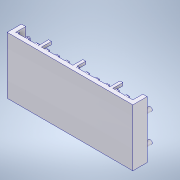
# Autodesk Inventor part: grip_4
Saved by Autodesk Inventor 2020 (Build 240168000, 168)
## iProperties
Created: 2019-10-09
Part Number: grip_4
Material: Generic
Document SubType Name: Modeling
Designer: ayad493
Density: 1 g/cm^3
Appearance: Cool White
Author: ayad493
Autodesk Inventor part; units mm, degrees
ref_plane "YZ Plane" through (0, 0, 0) normal (1, 0, 0) x (0, 1, 0)
ref_plane "XZ Plane" through (0, 0, 0) normal (0, 1, 0) x (-1, 0, 0)
ref_plane "XY Plane" through (0, 0, 0) normal (0, 0, 1) x (1, 0, 0)
sketch "Sketch1" plane through (0, 0, 0) normal (0, 0, 1) x (1, 0, 0)
  circle A0 centre (0, 0) radius 4
  arc A1 (0, 8) -> (0, -8) centre (0, 0) ccw
  circle A2 centre (60, 0) radius 4
  arc A3 (60, -8) -> (60, 8) centre (60, 0) ccw
  line L0 (0, 0) -> (4, 0)
  line L1 (60, 0) -> (45, 0)
  line L2 (15, 0) -> (15, -3.325)
  line L3 (45, 0) -> (45, -3.325)
  circle A4 centre (15, -1.6625) radius 1.6625
  circle A5 centre (45, -1.6625) radius 1.6625
  line L4 (0, -8) -> (60, -8)
  line L5 (0, 0) -> (0, 4)
  line L6 (0, 8) -> (30, 0)
  line L7 (30, 0) -> (60, 8)
  line L8 (0, 0) -> (15, 0)
  line L9 (45, 0) -> (60, 0)
  dimension "d0" = 8
  dimension "d1" = 16
  dimension "d2" = 60
  dimension "d3" = 8
  dimension "d4" = 16
  dimension "d5" = 3.325
  dimension "d63" = 60
  constraints: 20 end point, 6 point on circle, 4 centre point, 4 coincident, 3 horizontal, 2 midpoint, 2 vertical, 2 vertical alignment, 1 perpendicular, 1 tangent, 4 other
  measures "d0" diameter of A0
  measures "d1" diameter of A1
  measures "d2" distance of L0.start L9.end
  measures "d3" diameter of A2
  measures "d4" diameter of A3
  measures "d5" distance of L2.start L2.end
  measures "d63" distance of L4.start L4.end
extrude "Extrusion1" add sketch "Sketch1" along normal blind 20
fillet "Fillet2" radius 2 1 edges at (30, 0, 10)
sketch "Sketch20" plane through (0, -8, 0) normal (0, -1, 0) x (1, 0, 0)
  line L0 (60, 0) -> (60, 20) projected
  line L1 (60, 10) -> (52, 10)
  line L2 (52, 10) -> (52, 15)
  line L3 (-8, 0) -> (-8, 20) projected
  line L4 (52, 15) -> (-8, 15)
  line L5 (-8, 15) -> (-8, 5)
  line L6 (-8, 5) -> (52, 5)
  line L7 (52, 5) -> (52, 15)
  point P0 (0, 0)
  dimension "d65" = 5
  constraints: 12 end point, 2 horizontal, 2 parallel, 2 perpendicular, 1 midpoint, 1 point on line
  measures "d65" distance of L1.end L2.end
extrude "Extrusion18" cut sketch "Sketch20" against normal blind 20
sketch "Sketch21" plane through (0, -8, 0) normal (0, -1, 0) x (1, 0, 0)
  line L0 (0, 15) -> (0, 20) projected
  line L1 (0, 15) -> (8, 15)
  line L2 (-4, 15) -> (4, 15) projected
  line L3 (8, 15) -> (8, 5)
  line L4 (52, 5) -> (0, 5) projected
  line L5 (8, 15) -> (52, 15)
  line L6 (52, 15) -> (52, 5)
  line L7 (52, 5) -> (8, 5)
  line L8 (8, 5) -> (8, 15)
  constraints: 12 end point, 3 equal length, 2 perpendicular, 1 horizontal
extrude "Extrusion20" add sketch "Sketch21" against normal blind 4
sketch "Sketch22" plane through (0, 0, 20) normal (0, 0, 1) x (1, 0, 0)
  line L0 (52, -4) -> (8, -4) projected
  line L1 (8, -4) -> (10, -4)
  line L2 (10, -8) -> (10, -4)
  line L3 (10, -4) -> (10, -5)
  line L4 (10, -5) -> (52, -5)
  line L5 (52, -5) -> (52, -7)
  line L6 (52, -7) -> (10, -7)
  line L7 (10, -7) -> (10, -5)
  point P0 (0, 0)
  constraints: 14 end point, 2 parallel, 2 perpendicular, 2 point on line, 1 horizontal
extrude "Extrusion21" cut sketch "Sketch22" against normal blind 20
sketch "Sketch23" plane through (0, -8, 0) normal (0, -1, 0) x (1, 0, 0)
  line L0 (8, 5) -> (52, 5) projected
  line L1 (52, 15) -> (8, 15) projected
  line L2 (8, 15) -> (8, 5)
  line L3 (8, 5) -> (8, 15) projected
  circle A0 centre (13.5, 7.5) radius 1.5
  circle A1 centre (13.5, 12.5) radius 1.5
  circle A2 centre (23.5, 7.5) radius 1.5
  circle A3 centre (23.5, 12.5) radius 1.5
  circle A4 centre (33.5, 7.5) radius 1.5
  circle A5 centre (33.5, 12.5) radius 1.5
  circle A6 centre (43.5, 7.5) radius 1.5
  circle A7 centre (43.5, 12.5) radius 1.5
  line L4 (13.5, 12.5) -> (13.5, 17.5)
  line L5 (13.3375, 15) -> (13.3375, 20) projected
  line L6 (12, 16) -> (15, 16)
  line L7 (15, 16) -> (15, 19)
  line L8 (15, 19) -> (12, 19)
  line L9 (12, 19) -> (12, 16)
  line L10 (12, 16) -> (15, 19) construction
  line L11 (15, 16) -> (12, 19) construction
  line L12 (25, 19) -> (22, 19)
  line L13 (25, 16) -> (25, 19)
  line L14 (22, 19) -> (22, 16)
  line L15 (22, 16) -> (25, 16)
  line L16 (35, 19) -> (32, 19)
  line L17 (35, 16) -> (35, 19)
  line L18 (32, 19) -> (32, 16)
  line L19 (32, 16) -> (35, 16)
  line L20 (45, 19) -> (42, 19)
  line L21 (45, 16) -> (45, 19)
  line L22 (42, 19) -> (42, 16)
  line L23 (42, 16) -> (45, 16)
  line L24 (15, 14) -> (12, 14)
  line L25 (15, 11) -> (15, 14)
  line L26 (12, 14) -> (12, 11)
  line L27 (12, 11) -> (15, 11)
  line L28 (25, 14) -> (22, 14)
  line L29 (25, 11) -> (25, 14)
  line L30 (22, 14) -> (22, 11)
  line L31 (22, 11) -> (25, 11)
  line L32 (35, 14) -> (32, 14)
  line L33 (35, 11) -> (35, 14)
  line L34 (32, 14) -> (32, 11)
  line L35 (32, 11) -> (35, 11)
  line L36 (45, 14) -> (42, 14)
  line L37 (45, 11) -> (45, 14)
  line L38 (42, 14) -> (42, 11)
  line L39 (42, 11) -> (45, 11)
  line L40 (15, 9) -> (12, 9)
  line L41 (15, 6) -> (15, 9)
  line L42 (12, 9) -> (12, 6)
  line L43 (12, 6) -> (15, 6)
  line L44 (25, 9) -> (22, 9)
  line L45 (25, 6) -> (25, 9)
  line L46 (22, 9) -> (22, 6)
  line L47 (22, 6) -> (25, 6)
  line L48 (35, 9) -> (32, 9)
  line L49 (35, 6) -> (35, 9)
  line L50 (32, 9) -> (32, 6)
  line L51 (32, 6) -> (35, 6)
  line L52 (45, 9) -> (42, 9)
  line L53 (45, 6) -> (45, 9)
  line L54 (42, 9) -> (42, 6)
  line L55 (42, 6) -> (45, 6)
  line L56 (15, 4) -> (12, 4)
  line L57 (15, 1) -> (15, 4)
  line L58 (12, 4) -> (12, 1)
  line L59 (12, 1) -> (15, 1)
  line L60 (25, 4) -> (22, 4)
  line L61 (25, 1) -> (25, 4)
  line L62 (22, 4) -> (22, 1)
  line L63 (22, 1) -> (25, 1)
  line L64 (35, 4) -> (32, 4)
  line L65 (35, 1) -> (35, 4)
  line L66 (32, 4) -> (32, 1)
  line L67 (32, 1) -> (35, 1)
  line L68 (45, 4) -> (42, 4)
  line L69 (45, 1) -> (45, 4)
  line L70 (42, 4) -> (42, 1)
  line L71 (42, 1) -> (45, 1)
  point P0 (0, 0)
  dimension "d76" = 5
  dimension "d79" = 10
  dimension "d172" = 5
  dimension "d174" = 3
  dimension "d175" = 3
  dimension "d178" = 10
  dimension "d181" = 5
  constraints: 136 end point, 8 centre point, 3 horizontal, 3 parallel, 2 midpoint, 2 vertical, 1 perpendicular, 134 other
  measures "d76" distance of A0.centre L4.start
  measures "d79" distance of A0.centre A2.centre
  measures "d172" distance of L4.start L4.end
  measures "d174" distance of L8.end L7.end
  measures "d175" distance of L7.end L6.end
  measures "d178" distance of L7.end L12.start
  measures "d181" distance of L7.end L24.start
sketch "Sketch24" plane through (0, -8, 0) normal (0, -1, 0) x (1, 0, 0)
  circle A0 centre (13.5, 7.5) radius 1.5 projected
  circle A1 centre (23.5, 12.5) radius 1.5 projected
  line L0 (13.5, 7.5) -> (23.5, 12.5)
  circle A2 centre (33.5, 7.5) radius 1.5 projected
  line L1 (23.5, 12.5) -> (33.5, 7.5)
  circle A3 centre (43.5, 12.5) radius 1.5 projected
  line L2 (33.5, 7.5) -> (43.5, 12.5)
  line L3 (20, 8.5) -> (17, 8.5)
  line L4 (17, 8.5) -> (17, 11.5)
  line L5 (17, 11.5) -> (20, 11.5)
  line L6 (20, 11.5) -> (20, 8.5)
  line L7 (20, 8.5) -> (17, 11.5) construction
  line L8 (17, 8.5) -> (20, 11.5) construction
  line L9 (27, 8.5) -> (30, 8.5)
  line L10 (30, 8.5) -> (30, 11.5)
  line L11 (30, 11.5) -> (27, 11.5)
  line L12 (27, 11.5) -> (27, 8.5)
  line L13 (27, 8.5) -> (30, 11.5) construction
  line L14 (30, 8.5) -> (27, 11.5) construction
  line L15 (40, 8.5) -> (37, 8.5)
  line L16 (37, 8.5) -> (37, 11.5)
  line L17 (37, 11.5) -> (40, 11.5)
  line L18 (40, 11.5) -> (40, 8.5)
  line L19 (40, 8.5) -> (37, 11.5) construction
  line L20 (37, 8.5) -> (40, 11.5) construction
  circle A4 centre (13.5, 12.5) radius 1.5 projected
  line L21 (13.5, 7.5) -> (13.5, 12.5)
  line L22 (13.5, 12.5) -> (13.5, 20)
  line L23 (13.5, 15) -> (13.5, 20)
  line L24 (0, 20) -> (60, 20) projected
  line L25 (12, 16) -> (15, 16)
  line L26 (15, 16) -> (15, 19)
  line L27 (15, 19) -> (12, 19)
  line L28 (12, 19) -> (12, 16)
  line L29 (12, 16) -> (15, 19) construction
  line L30 (15, 16) -> (12, 19) construction
  line L31 (12, 4) -> (12, 1)
  line L32 (12, 1) -> (15, 1)
  line L33 (15, 1) -> (15, 4)
  line L34 (15, 4) -> (12, 4)
  line L35 (22, 19) -> (22, 16)
  line L36 (22, 16) -> (25, 16)
  line L37 (25, 16) -> (25, 19)
  line L38 (25, 19) -> (22, 19)
  line L39 (22, 4) -> (22, 1)
  line L40 (22, 1) -> (25, 1)
  line L41 (25, 1) -> (25, 4)
  line L42 (25, 4) -> (22, 4)
  line L43 (32, 19) -> (32, 16)
  line L44 (32, 16) -> (35, 16)
  line L45 (35, 16) -> (35, 19)
  line L46 (35, 19) -> (32, 19)
  line L47 (32, 4) -> (32, 1)
  line L48 (32, 1) -> (35, 1)
  line L49 (35, 1) -> (35, 4)
  line L50 (35, 4) -> (32, 4)
  line L51 (42, 19) -> (42, 16)
  line L52 (42, 16) -> (45, 16)
  line L53 (45, 16) -> (45, 19)
  line L54 (45, 19) -> (42, 19)
  line L55 (42, 4) -> (42, 1)
  line L56 (42, 1) -> (45, 1)
  line L57 (45, 1) -> (45, 4)
  line L58 (45, 4) -> (42, 4)
  point P0 (0, 0)
  point P1 (18.5, 10)
  point P2 (28.5, 10)
  point P3 (38.5, 10)
  point P4 (13.5, 17.5)
  dimension "d84" = 3
  dimension "d85" = 3
  dimension "d88" = 15
  dimension "d91" = 10
  constraints: 116 end point, 12 midpoint, 9 parallel, 5 horizontal, 5 perpendicular, 4 point on line, 2 vertical, 56 other
  measures "d84" distance of L3.end L4.end
  measures "d85" distance of L16.end L17.end
  measures "d88" distance of L27.end L31.start
  measures "d91" distance of L27.end L35.start
extrude "Extrusion23" add sketch "Sketch24" against normal blind 4 contours L4 L5 L6 L0 | L0 L6 L3 L4 | L12 L11 L10 L1 | L1 L10 L9 L12 | L16 L17 L18 L2 | L2 L18 L15 L16 | L25 L28 L27 L22 | L22 L27 L26 L25 | L34 L33 L32 L31 | L38 L37 L36 L35 | L42 L41 L40 L39 | L46 L45 L44 L43 | L50 L49 L48 L47 | L54 L53 L52 L51 | L58 L57 L56 L55
sketch "Sketch25" plane through (0, -8, 0) normal (0, -1, 0) x (1, 0, 0)
  line L0 (68, 0) -> (68, 20) projected
  line L1 (68, 0) -> (52, 0)
  line L2 (52, 0) -> (52, 6)
  line L3 (52, 6) -> (68, 6)
  line L4 (68, 6) -> (68, 0)
  line L5 (68, 20) -> (60, 20) projected
  line L6 (68, 20) -> (52, 20)
  line L7 (52, 20) -> (52, 14)
  line L8 (52, 14) -> (68, 14)
  line L9 (68, 14) -> (68, 20)
  point P0 (0, 0)
  constraints: 16 end point, 4 parallel, 2 horizontal, 2 perpendicular, 2 point on line
extrude "Extrusion24" cut sketch "Sketch25" against normal blind 18
sketch "Sketch26" plane through (0, -8, 15) normal (0, -1, 0) x (1, 0, 0)
  line L0 (52, -15) -> (30.5153, -15) projected
  line L1 (52, -15) -> (50, -15)
  line L2 (50, -15) -> (50, 5)
  line L3 (50, 5) -> (52, 5)
  line L4 (52, 5) -> (52, -15)
  point P0 (0, -15)
  constraints: 8 end point, 2 parallel, 1 horizontal, 1 perpendicular
extrude "Extrusion25" add sketch "Sketch26" against normal blind 16
sketch "Sketch27" plane through (0, 0, 0) normal (0, 0, -1) x (-1, 0, 0)
  line L0 (-52, -8) -> (-52, 5.8667) projected
  line L1 (-50, -4) -> (-50, 5.3333) projected
  line L2 (-52, 5.8667) -> (-50, 5.3333)
  line L3 (-50, 5.3333) -> (-50, 8)
  line L4 (-52, 8) -> (-50, 8) projected
  line L5 (-50, 8) -> (-52, 8)
  line L6 (-52, 8) -> (-52, 5.8667)
  line L7 (-52, 8) -> (-52, -8) projected
  point P0 (0, 0)
  constraints: 8 end point, 3 collinear
extrude "Extrusion26" cut sketch "Sketch27" against normal blind 20
fillet "Fillet3" radius 2 3 edges at (60, 8, 10) (0, 8, 2.5) (0, 8, 17.5)
sketch "Sketch28" plane through (60, -8, 6) normal (0, 0, -1) x (-1, 0, 0)
  line L0 (0, 0) -> (8, 0) projected
  line L1 (0, 0) -> (0, 1)
  circle A0 centre (15, 6.3375) radius 1.6625 projected
  line L2 (15, 6.3375) -> (15, 8)
  arc A1 (-0.3247, 15.9934) -> (0, 0) centre (0, 8) ccw projected
  arc A2 (-5.6569, 13.6569) -> (5, 1.755) centre (0, 8) ccw
  line L3 (10, 5.0386) -> (5, 1.755)
  arc A3 (-4.773, 12.773) -> (4.1504, 2.6768) centre (0, 8) ccw
  line L4 (15, 8) -> (15, 9.5)
  line L5 (15, 9.5) -> (4.1504, 2.6768)
  line L6 (10, 4) -> (10, 13.3333) projected
  line L7 (10, 6.3555) -> (10, 5.0386)
  line L8 (-4.773, 12.773) -> (-5.6569, 13.6569)
  line L9 (0, 8) -> (8, 8) construction
  line L10 (8, 0) -> (0, 0) projected
  line L11 (0, 0) -> (8, 0)
  line L12 (8, 0) -> (8, 3.7252)
  line L13 (8, 13.8667) -> (8, 0) projected
  point P0 (60, 8)
  dimension "d103" = 13.5
  dimension "d104" = 1.5
  dimension "d105" = 135
  constraints: 20 end point, 5 point on circle, 5 point on line, 3 vertical, 2 centre point, 2 coincident, 1 collinear, 1 horizontal, 1 vertical alignment, 1 other
  measures "d103" diameter of A3
  measures "d104" distance of L2.end L4.end
  measures "d105" angle of L9 L8
extrude "Extrusion29" cut sketch "Sketch28" against normal blind 5 contours A2 L3 L12 L0 | A1 L8 A3 L5 L13 L3 A2 | L13 L5 L6 L3
sketch "Sketch30" plane through (52, -2.9022, 6) normal (0, 0, -1) x (-1, 0, 0)
  circle A0 centre (-8, 2.9022) radius 4 projected
  arc A1 (-13.6569, 8.5591) -> (-8, -5.0978) centre (-8, 2.9022) ccw
  arc A2 (-12.773, 7.6752) -> (-3.8496, -2.421) centre (-8, 2.9022) ccw
  line L0 (0, -5.0978) -> (0, 8.7689) projected
  line L1 (-3.8496, -2.421) -> (2, 1.2578) projected
  line L2 (0, 0) -> (-0.7447, -0.4683)
  line L3 (-8, -5.0978) -> (0, -5.0978) projected
  line L4 (0, 0) -> (0, -5.0978)
  line L5 (0, -5.0978) -> (-8, -5.0978)
  line L6 (-13.6569, 8.5591) -> (-12.773, 7.6752) projected
  line L7 (-12.773, 7.6752) -> (-13.6569, 8.5591)
  line L8 (0, -1.3726) -> (0, 0) projected
  line L9 (0, -1.3726) -> (2, -0.0592) projected
  line L10 (0, -1.3726) -> (2, -0.0592)
  line L11 (2, 1.2578) -> (2, -0.0592) projected
  line L12 (2, -0.0592) -> (2, 1.2578)
  line L13 (2, 1.2578) -> (0, 0) projected
  line L14 (2, 1.2578) -> (0, 0)
  line L15 (0, 0) -> (0, -1.3726)
  point P0 (52, 2.9022)
  constraints: 18 end point, 6 collinear, 5 point on circle, 4 point on line, 2 centre point, 2 coincident, 1 vertical
extrude "Extrusion33" add sketch "Sketch30" against normal blind 3 contours L6 A2 L1 L0 L3 A1 | L0 L1 L11 L9
fillet "Fillet4" radius 2 1 edges at (64.773, 4.773, 10)
fillet "Fillet5" radius 2 1 edges at (52, -4.2748, 10)
sketch "Sketch31" plane through (0, -8, 15) normal (0, -1, 0) x (1, 0, 0)
  line L0 (52, -15) -> (52, -9) projected
  line L1 (10, 5) -> (10, -15) projected
  line L2 (52, -15) -> (10, -15)
  line L3 (10, -15) -> (10, -12)
  line L4 (10, -12) -> (52, -12)
  line L5 (52, -12) -> (52, -15)
  line L6 (52, 5) -> (10, 5)
  line L7 (10, 5) -> (10, 2)
  line L8 (10, 2) -> (52, 2)
  line L9 (52, 2) -> (52, 5)
  point P0 (0, -15)
  constraints: 16 end point, 4 parallel, 3 point on line, 2 horizontal, 2 perpendicular
extrude "Extrusion34" add sketch "Sketch31" against normal blind 3
sketch "Sketch32" plane through (8, -8, 5) normal (-1, 0, 0) x (0, 0, 1)
  line L0 (6, 1.25) -> (4, 1.25) projected
  line L1 (6, 2.6459) -> (4, 2.6459) projected
  line L2 (6, 1.25) -> (4, 2.6459)
  circle A0 centre (5, 1.9479) radius 0.75
  point P0 (-5, 8)
  dimension "d124" = 1.5
  constraints: 2 end point, 1 centre point, 1 midpoint, 1 point on line
  measures "d124" diameter of A0
extrude "Extrusion35" cut sketch "Sketch32" against normal blind 3 contours A0 L0 | L0 A0 L2 | L2 A0 L1 | A0 L1 picked at (5.0916, 1.7153) picked at (5.0915, 2.1806)
sketch "Sketch33" plane through (0, 0, 20) normal (0, 0, 1) x (1, 0, 0)
  line L0 (0, -8) -> (52, -8) projected
  line L1 (8, -8) -> (8, -14)
  line L2 (8, -14) -> (50, -14)
  line L3 (52, -12) -> (52, -8)
  line L4 (52, -8) -> (51.5, -8)
  line L5 (51.5, -8) -> (51.5, -10.5)
  line L6 (49.5, -12.5) -> (8.5, -12.5) construction
  line L7 (8.5, -12.5) -> (8.5, -8)
  arc A0 (49.5, -12.5) -> (51.5, -10.5) centre (49.5, -10.5) ccw
  arc A1 (50, -14) -> (52, -12) centre (50, -12) ccw
  line L8 (49, -12) -> (49.5, -12.5)
  line L9 (49, -12) -> (48.5, -12.5)
  line L10 (48.5, -12.5) -> (48, -12)
  line L11 (48, -12) -> (47.5, -12.5)
  line L12 (47, -12) -> (47.5, -12.5)
  line L13 (47, -12) -> (46.5, -12.5)
  line L14 (46.5, -12.5) -> (46, -12)
  line L15 (46, -12) -> (45.5, -12.5)
  line L16 (45, -12) -> (45.5, -12.5)
  line L17 (45, -12) -> (44.5, -12.5)
  line L18 (44.5, -12.5) -> (44, -12)
  line L19 (44, -12) -> (43.5, -12.5)
  line L20 (43, -12) -> (43.5, -12.5)
  line L21 (43, -12) -> (42.5, -12.5)
  line L22 (42.5, -12.5) -> (42, -12)
  line L23 (42, -12) -> (41.5, -12.5)
  line L24 (41, -12) -> (41.5, -12.5)
  line L25 (41, -12) -> (40.5, -12.5)
  line L26 (40.5, -12.5) -> (40, -12)
  line L27 (40, -12) -> (39.5, -12.5)
  line L28 (39, -12) -> (39.5, -12.5)
  line L29 (39, -12) -> (38.5, -12.5)
  line L30 (38.5, -12.5) -> (38, -12)
  line L31 (38, -12) -> (37.5, -12.5)
  line L32 (37, -12) -> (37.5, -12.5)
  line L33 (37, -12) -> (36.5, -12.5)
  line L34 (36.5, -12.5) -> (36, -12)
  line L35 (36, -12) -> (35.5, -12.5)
  line L36 (35, -12) -> (35.5, -12.5)
  line L37 (35, -12) -> (34.5, -12.5)
  line L38 (34.5, -12.5) -> (34, -12)
  line L39 (34, -12) -> (33.5, -12.5)
  line L40 (33, -12) -> (33.5, -12.5)
  line L41 (33, -12) -> (32.5, -12.5)
  line L42 (32.5, -12.5) -> (32, -12)
  line L43 (32, -12) -> (31.5, -12.5)
  line L44 (31, -12) -> (31.5, -12.5)
  line L45 (31, -12) -> (30.5, -12.5)
  line L46 (30.5, -12.5) -> (30, -12)
  line L47 (30, -12) -> (29.5, -12.5)
  line L48 (29, -12) -> (29.5, -12.5)
  line L49 (29, -12) -> (28.5, -12.5)
  line L50 (28.5, -12.5) -> (28, -12)
  line L51 (28, -12) -> (27.5, -12.5)
  line L52 (27, -12) -> (27.5, -12.5)
  line L53 (27, -12) -> (26.5, -12.5)
  line L54 (26.5, -12.5) -> (26, -12)
  line L55 (26, -12) -> (25.5, -12.5)
  line L56 (25, -12) -> (25.5, -12.5)
  line L57 (25, -12) -> (24.5, -12.5)
  line L58 (24.5, -12.5) -> (24, -12)
  line L59 (24, -12) -> (23.5, -12.5)
  line L60 (23, -12) -> (23.5, -12.5)
  line L61 (23, -12) -> (22.5, -12.5)
  line L62 (22.5, -12.5) -> (22, -12)
  line L63 (22, -12) -> (21.5, -12.5)
  line L64 (21, -12) -> (21.5, -12.5)
  line L65 (21, -12) -> (20.5, -12.5)
  line L66 (20.5, -12.5) -> (20, -12)
  line L67 (20, -12) -> (19.5, -12.5)
  line L68 (19, -12) -> (19.5, -12.5)
  line L69 (19, -12) -> (18.5, -12.5)
  line L70 (18.5, -12.5) -> (18, -12)
  line L71 (18, -12) -> (17.5, -12.5)
  line L72 (17, -12) -> (17.5, -12.5)
  line L73 (17, -12) -> (16.5, -12.5)
  line L74 (16.5, -12.5) -> (16, -12)
  line L75 (16, -12) -> (15.5, -12.5)
  line L76 (15, -12) -> (15.5, -12.5)
  line L77 (15, -12) -> (14.5, -12.5)
  line L78 (14.5, -12.5) -> (14, -12)
  line L79 (14, -12) -> (13.5, -12.5)
  line L80 (13, -12) -> (13.5, -12.5)
  line L81 (13, -12) -> (12.5, -12.5)
  line L82 (12.5, -12.5) -> (12, -12)
  line L83 (12, -12) -> (11.5, -12.5)
  line L84 (11, -12) -> (11.5, -12.5)
  line L85 (11, -12) -> (10.5, -12.5)
  line L86 (10.5, -12.5) -> (10, -12)
  line L87 (10, -12) -> (9.5, -12.5)
  line L88 (49.5, -12.5) -> (49, -12)
  line L89 (48.5, -12.5) -> (48, -12)
  line L90 (47.5, -12.5) -> (47, -12)
  line L91 (46.5, -12.5) -> (46, -12)
  line L92 (45.5, -12.5) -> (45, -12)
  line L93 (44.5, -12.5) -> (44, -12)
  line L94 (43.5, -12.5) -> (43, -12)
  line L95 (42.5, -12.5) -> (42, -12)
  line L96 (41.5, -12.5) -> (41, -12)
  line L97 (40.5, -12.5) -> (40, -12)
  line L98 (39.5, -12.5) -> (39, -12)
  line L99 (38.5, -12.5) -> (38, -12)
  line L100 (38, -12) -> (37.5, -12.5)
  line L101 (37, -12) -> (36.5, -12.5)
  line L102 (36, -12) -> (35.5, -12.5)
  line L103 (35, -12) -> (34.5, -12.5)
  line L104 (34, -12) -> (33.5, -12.5)
  line L105 (33, -12) -> (32.5, -12.5)
  line L106 (32, -12) -> (31.5, -12.5)
  line L107 (31, -12) -> (30.5, -12.5)
  line L108 (30, -12) -> (29.5, -12.5)
  line L109 (29, -12) -> (28.5, -12.5)
  line L110 (28, -12) -> (27.5, -12.5)
  line L111 (27, -12) -> (26.5, -12.5)
  line L112 (26, -12) -> (25.5, -12.5)
  line L113 (25, -12) -> (24.5, -12.5)
  line L114 (24, -12) -> (23.5, -12.5)
  line L115 (23, -12) -> (22.5, -12.5)
  line L116 (22, -12) -> (21.5, -12.5)
  line L117 (21, -12) -> (20.5, -12.5)
  line L118 (20, -12) -> (19.5, -12.5)
  line L119 (19, -12) -> (18.5, -12.5)
  line L120 (18, -12) -> (17.5, -12.5)
  line L121 (17, -12) -> (16.5, -12.5)
  line L122 (16, -12) -> (15.5, -12.5)
  line L123 (15, -12) -> (14.5, -12.5)
  line L124 (14, -12) -> (13.5, -12.5)
  line L125 (13, -12) -> (12.5, -12.5)
  line L126 (12, -12) -> (11.5, -12.5)
  line L127 (11, -12) -> (10.5, -12.5)
  line L128 (10, -12) -> (9.5, -12.5)
  line L129 (9.5, -12.5) -> (8.5, -12.5)
  line L130 (52, -8) -> (51.5, -8)
  line L131 (8.5, -8) -> (8, -8)
  line L132 (52, -8) -> (52, 5.8667) projected
  line L133 (52, -12) -> (52, -8)
  line L134 (52, -8) -> (51.5, -8)
  line L135 (52, -8) -> (51.5, -8)
  line L136 (9.5, -12.5) -> (8.5, -12.5)
  line L137 (8.5, -14) -> (49.5, -14)
  line L138 (49.5, -14) -> (49.5, -12.5)
  arc A2 (50, -14) -> (52, -12) centre (50, -12) ccw
  line L139 (8, -14) -> (8.5, -14)
  line L140 (8.5, -12.5) -> (8.5, -8)
  line L141 (8.5, -8) -> (8, -8)
  line L142 (8, -8) -> (8, -14)
  line L143 (0, -8) -> (52, -8) projected
  line L144 (51.5, -8) -> (52, -8)
  line L145 (52, -8) -> (52, -12)
  line L146 (51.5, -8) -> (51.5, -10.5)
  point P0 (0, 0)
  point P1 (51.5, -12.5)
  dimension "d129" = 43
  dimension "d130" = 2
  dimension "d134" = 2
  dimension "d139" = 0.5
  dimension "d140" = 0.5
  dimension "d158" = 4.5
  dimension "d159" = 6
  dimension "d160" = 2.5
  constraints: 289 end point, 32 collinear, 22 coincident, 14 perpendicular, 12 parallel, 6 point on circle, 6 point on line, 5 horizontal, 5 tangent, 3 centre point, 1 equal radius, 1 vertical, 190 other
  measures "d129" distance of L6.end point (51.5, -12.5)
  measures "d130" radius of A0
  measures "d134" distance of L6.start point (47.5, -12.5)
  measures "d139" horizontal distance of L9.end L8.start
  measures "d140" horizontal distance of L9.end L10.end
  measures "d158" distance of L6.end L7.end
  measures "d159" distance of L1.start L1.end
  measures "d160" distance of L4.end L5.end
extrude "Extrusion36" add sketch "Sketch33" against normal blind 20 contours L0 L7 L129 L87 L86 L85 L84 L83 L82 L81 L80 L79 L78 L77 L76 L75 L74 L73 L72 L71 L70 L69 L68 L67 L66 L65 L64 L63 L62 L61 L60 L59 L58 L57 L56 L55 L54 L53 L52 L51 L50 L49 L48 L47 L46 L45 L44 L43 L42 L41 L40 L39 L38 L37 L36 L35 L34 L33 L32 L31 L30 L29 L28 L27 L26 L25 L24 L23 L22 L21 L20 L19 L18 L17 L16 L15 L14 L13 L12 L11 L10 L9 L8 L138 L2 L1
sketch "Sketch35" plane through (0, 0, 20) normal (0, 0, 1) x (1, 0, 0)
  line L0 (52, 5.8667) -> (52, -8) projected
  line L1 (52, -8) -> (51.5, -8)
  line L2 (51.5, -8) -> (51.5, -14)
  line L3 (51.5, -14) -> (52, -14)
  line L4 (52, -14) -> (52, -8)
  line L5 (49.5, -14) -> (8, -14) projected
  line L6 (49.5, -14) -> (52, -14)
  line L7 (52, -14) -> (52, -13.5)
  line L8 (52, -13.5) -> (49.5, -13.5)
  line L9 (49.5, -13.5) -> (49.5, -14)
  point P0 (0, 0)
  point P1 (51.5, -13.5)
  dimension "d143" = 0.5
  dimension "d144" = 0.5
  dimension "d161" = 6
  constraints: 16 end point, 4 parallel, 2 horizontal, 2 perpendicular, 1 point on line
  measures "d143" distance of L3.end L2.end
  measures "d144" distance of L7.end L6.end
  measures "d161" distance of L3.end L0.end
sketch "Sketch36" plane through (8, -8, 0) normal (-1, 0, 0) x (0, 0, 1)
  line L0 (0, -1.5) -> (1.4518, -1.5)
  circle A0 centre (10, 1.9479) radius 0.75 projected
  line L1 (1.4518, -1.5) -> (10, -1.5)
  circle A1 centre (10, 1.9479) radius 0.75 projected
  line L2 (10, 1.9479) -> (10, -1.5)
  line L3 (10, -1.5) -> (10, -2)
  circle A2 centre (10, -2) radius 1.75
  point P0 (0, 8)
  dimension "d166" = 0.5
  dimension "d167" = 3.5
  constraints: 8 end point, 2 vertical, 1 centre point, 1 coincident, 1 horizontal
  measures "d166" distance of L1.end L3.end
  measures "d167" diameter of A2
sketch "Sketch37" plane through (0, 0, 20) normal (0, 0, 1) x (1, 0, 0)
  circle A0 centre (0, 0) radius 4
  circle A1 centre (0, 0) radius 3
  dimension "d150" = 6
  constraints: 2 centre point, 2 coincident
  measures "d150" diameter of A1
extrude "Extrusion39" add sketch "Sketch37" against normal blind 5
sketch "Sketch38" plane through (0, 0, 0) normal (0, 0, -1) x (-1, 0, 0)
  circle A0 centre (0, 0) radius 4
  circle A1 centre (0, 0) radius 3
  constraints: 2 centre point, 2 coincident
extrude "Extrusion40" add sketch "Sketch38" against normal blind 5
sketch "Sketch39" plane through (60, -8, 6) normal (0, 0, -1) x (-1, 0, 0)
  circle A0 centre (0, 8) radius 4 projected
  circle A1 centre (0, 8) radius 4
  circle A2 centre (0, 8) radius 3
  point P0 (60, 8)
  dimension "d155" = 6
  constraints: 2 centre point, 2 coincident
  measures "d155" diameter of A2
extrude "Extrusion41" add sketch "Sketch39" against normal up to surface (8 mm away)
extrude "Extrusion42" add sketch "Sketch35" against normal up to surface (20 mm away)
fillet "Fillet7" radius 3 2 edges at (52, -14, 10) (51.5, -13.5, 10)
extrude "Extrusion43" cut sketch "Sketch36" against normal blind 2 contours A2 L2 L1 | L1 L2 A2
sketch "Sketch40" plane through (0, 0, 0) normal (0, 0, -1) x (-1, 0, 0)
  line L0 (-49.5, -12.5) -> (-49, -12) projected
  line L1 (-49.5, -12.5) -> (-50.8784, -12.5)
  arc A0 (-51.5, -10.6716) -> (-49.5, -13.5) centre (-48.5, -10.6716) ccw projected
  line L2 (-49.5, -13.5) -> (-49.5, -12.5)
  arc A1 (-50.8784, -12.5) -> (-49.5, -13.5) centre (-48.5, -10.6716) ccw
  point P0 (0, 0)
  constraints: 4 end point, 3 point on circle, 1 centre point, 1 concentric, 1 horizontal, 1 perpendicular
extrude "Extrusion44" add sketch "Sketch40" against normal up to surface (20 mm away)
extrude "Extrusion45" cut sketch "Sketch23" against normal blind 2 contours L6 L5 L8 L7 | L6 L9 L8 L5 | A0 | L41 L43 A0 | A0 L40 L41 | A0 L42 L40 | L43 L42 A0 | A1 | L25 L27 A1 | A1 L24 L25 | A1 L26 L24 | L27 L26 A1 | A2 | L45 L47 A2 | A2 L44 L45 | A2 L46 L44 | L47 L46 A2 | A3 | L29 L31 A3 | A3 L28 L29 | A3 L30 L28 | L31 L30 A3 | A4 | L49 L51 A4 | A4 L48 L49 | A4 L50 L48 | L51 L50 A4 | A5 | L33 L35 A5 | A5 L32 L33 | A5 L34 L32 | L35 L34 A5 | A6 | L53 L55 A6 | A6 L52 L53 | A6 L54 L52 | L55 L54 A6 | A7 | L37 L39 A7 | A7 L36 L37 | A7 L38 L36 | L39 L38 A7 | L13 L15 L14 L12 | L17 L19 L18 L16 | L21 L23 L22 L20 | L57 L59 L58 L56 | L61 L63 L62 L60 | L65 L67 L66 L64 | L69 L71 L70 L68
sketch "Sketch41" plane through (0, 0, 20) normal (0, 0, 1) x (1, 0, 0)
  line L0 (8.5, -8) -> (51.5, -8) projected
  line L1 (51.5, -8) -> (8.5, -8)
  line L2 (8.5, -12.5) -> (8.5, -8) projected
  line L3 (8.5, -8) -> (8.5, -12.5)
  line L4 (8.5, -12.5) -> (8.5, -10.25)
  line L5 (51.5, -10.25) -> (8.5, -10.25)
  line L6 (29.5, -8) -> (30.5, -8)
  line L7 (30.5, -8) -> (30.5, -12.5)
  line L8 (30.5, -12.5) -> (29.5, -12.5)
  line L9 (29.5, -12.5) -> (29.5, -8)
  line L10 (29.5, -8) -> (30.5, -12.5) construction
  line L11 (30.5, -8) -> (29.5, -12.5) construction
  line L12 (43, -12) -> (43, -8)
  line L13 (45, -8) -> (42, -8) projected
  line L14 (18, -12) -> (18, -8)
  line L15 (42.5, -12.5) -> (42, -12) projected
  line L16 (43.5, -8) -> (42.5, -8)
  line L17 (42.5, -8) -> (42.5, -12.5)
  line L18 (42.5, -12.5) -> (43.5, -12.5)
  line L19 (43.5, -12.5) -> (43.5, -8)
  line L20 (43.5, -8) -> (42.5, -12.5) construction
  line L21 (42.5, -8) -> (43.5, -12.5) construction
  line L22 (17.5, -12.5) -> (18, -12) projected
  line L23 (18.5, -8) -> (17.5, -8)
  line L24 (17.5, -8) -> (17.5, -12.5)
  line L25 (17.5, -12.5) -> (18.5, -12.5)
  line L26 (18.5, -12.5) -> (18.5, -8)
  line L27 (18.5, -8) -> (17.5, -12.5) construction
  line L28 (17.5, -8) -> (18.5, -12.5) construction
  point P0 (0, 0)
  point P1 (30, -10.25)
  point P2 (43, -10.25)
  point P3 (18, -10.25)
  dimension "d186" = 1
  constraints: 48 end point, 8 midpoint, 7 perpendicular, 6 parallel, 6 point on line, 4 horizontal
  measures "d186" distance of L7.end L8.end
extrude "Extrusion46" add sketch "Sketch41" against normal blind 1 contours L0 L14 L5 L24 | L0 L26 L5 L14 | L5 L14 L22 L24 | L5 L26 L25 L22 L14 | L0 L7 L5 L9 | L5 L7 L8 L9 | L0 L12 L5 L17 | L5 L19 L18 L17 | L0 L19 L5 L12
sketch "Sketch42" plane through (0, 0, 0) normal (0, 0, -1) x (-1, 0, 0)
  line L0 (-18.5, -12.5) -> (-18.5, -8) projected
  line L1 (-17.5, -12.5) -> (-17.5, -8) projected
  line L2 (-18.5, -8) -> (-17.5, -8)
  line L3 (-17.5, -8) -> (-17.5, -12.5)
  line L4 (-17.5, -12.5) -> (-18.5, -12.5)
  line L5 (-18.5, -12.5) -> (-18.5, -8)
  line L6 (-29, -12) -> (-29.5, -12.5) projected
  line L7 (-30.5, -8) -> (-30.5, -12.5) projected
  line L8 (-29.5, -12.5) -> (-30.5, -12.5)
  line L9 (-30.5, -12.5) -> (-30.5, -8)
  line L10 (-30.5, -8) -> (-29.5, -8)
  line L11 (-29.5, -8) -> (-29.5, -12.5)
  line L12 (-42, -8) -> (-45, -8) projected
  line L13 (-42.5, -12.5) -> (-43.5, -12.5)
  line L14 (-43.5, -12.5) -> (-43.5, -8)
  line L15 (-43.5, -8) -> (-42.5, -8)
  line L16 (-42.5, -8) -> (-42.5, -12.5)
  point P0 (0, 0)
  constraints: 24 end point, 6 parallel, 3 horizontal, 3 perpendicular, 1 midpoint
extrude "Extrusion47" add sketch "Sketch42" against normal blind 1
sketch "Sketch43" plane through (0, 0, 20) normal (0, 0, 1) x (1, 0, 0)
  circle A0 centre (0, 0) radius 3 projected
  line L0 (0, 0) -> (-5.6569, 5.6569)
  arc A1 (-0.3247, 7.9934) -> (0, -8) centre (0, 0) ccw projected
  line L1 (0, 0) -> (8, 0) construction
  circle A2 centre (-5.6569, 5.6569) radius 2.5
  point P0 (-3.6346, 7.1267)
  point P1 (-7.1267, 3.6346)
  dimension "d191" = 135
  dimension "d192" = 5
  constraints: 4 end point, 1 centre point, 1 coincident, 1 equal length, 1 horizontal, 1 point on circle
  measures "d191" angle of L1 L0
  measures "d192" diameter of A2
extrude "Extrusion48" add sketch "Sketch43" against normal up to surface (20 mm away) contours A1 A2
sketch "Sketch44" plane through (29.4847, 0.1374, 5) normal (0.2576627, 0.9662349, 0) x (0.9662349, -0.2576627, 0)
  line L0 (-33.8019, -10) -> (-30.8271, -10) projected
  line L1 (-33.8019, -10) -> (-38.8019, -10)
  line L2 (-38.8019, -10) -> (-38.8019, 0)
  line L3 (-38.8019, 0) -> (-33.8019, 0)
  line L4 (-33.8019, 0) -> (-33.8019, -10)
  point P0 (-28.4537, 5)
  dimension "d195" = 5
  dimension "d196" = 10
  constraints: 8 end point, 2 parallel, 1 horizontal, 1 perpendicular
  measures "d195" distance of L2.end L3.end
  measures "d196" distance of L1.end L2.end
extrude "Extrusion49" cut sketch "Sketch44" against normal blind 10
sketch "Sketch45" plane through (30.5153, 0.1374, 5) normal (-0.2576627, 0.9662349, 0) x (0.9662349, 0.2576627, 0)
  line L0 (18.6625, -1) -> (22.2355, -1) projected
  line L1 (22.2355, -1) -> (22.2355, -9)
  line L2 (31.4537, -9) -> (25.4537, -9) projected
  line L3 (22.2355, -5) -> (26.2355, -5)
  line L4 (24.8855, -2.6) -> (27.6389, -2.6309)
  line L5 (27.6389, -2.6309) -> (28.9889, -5.0309)
  line L6 (28.9889, -5.0309) -> (27.5855, -7.4)
  line L7 (27.5855, -7.4) -> (24.832, -7.3691)
  line L8 (24.832, -7.3691) -> (23.482, -4.9691)
  line L9 (23.482, -4.9691) -> (24.8855, -2.6)
  point P0 (-29.5204, 5)
  dimension "d199" = 8
  dimension "d200" = 4
  constraints: 16 end point, 1 horizontal, 1 midpoint, 1 perpendicular, 13 other
  measures "d199" distance of L0.end L1.end
  measures "d200" distance of L3.start L3.end
extrude "Extrusion50" cut sketch "Sketch45" against normal blind 1.7
sketch "Sketch46" plane through (0, 0, 20) normal (0, 0, 1) x (1, 0, 0)
  line L0 (52, -8) -> (52, 5.8667) projected
  line L1 (52, -8) -> (50.5, -8)
  line L2 (50.5, -8) -> (50.5, -14)
  line L3 (50.5, -14) -> (52, -14)
  line L4 (52, -14) -> (52, -8)
  line L5 (8, -8) -> (8, -14) projected
  line L6 (8, -14) -> (49, -14) projected
  line L7 (8, -8) -> (9.5, -8)
  line L8 (9.5, -8) -> (9.5, -14)
  line L9 (9.5, -14) -> (8, -14)
  line L10 (8, -14) -> (8, -8)
  point P0 (0, 0)
  dimension "d205" = 1.5
  dimension "d206" = 1.5
  constraints: 16 end point, 4 parallel, 2 horizontal, 2 perpendicular, 1 point on line
  measures "d205" distance of L3.end L2.end
  measures "d206" distance of L8.end L9.end
extrude "Extrusion51" add sketch "Sketch46" against normal up to surface (20 mm away)
sketch "Sketch47" plane through (0, 0, 20) normal (0, 0, 1) x (1, 0, 0)
  line L0 (52, 5.8667) -> (52, -14) projected
  line L1 (8, -8) -> (8, -14) projected
  line L2 (52, -14) -> (8, -14)
  line L3 (8, -14) -> (8, -13.3004)
  line L4 (8, -13.3004) -> (52, -13.3004)
  line L5 (52, -13.3004) -> (52, -14)
  point P0 (0, 0)
  constraints: 8 end point, 2 parallel, 1 horizontal, 1 perpendicular, 1 point on line
extrude "Extrusion52" add sketch "Sketch47" against normal up to surface (20 mm away)
sketch "Sketch48" plane through (8, -14, 20) normal (0, -1, 0) x (1, 0, 0)
  line L0 (42.5, -20) -> (42.5, 0) projected
  line L1 (44, -20) -> (0, -20) projected
  line L2 (42.5, -20) -> (44, -20)
  line L3 (44, -20) -> (43.25, -20)
  line L4 (43.25, -14.25) -> (43.25, -15.75)
  line L5 (43.25, -5.75) -> (43.25, -4.25)
  line L6 (44, 0) -> (22.5153, 0) projected
  line L7 (44, -14.25) -> (42.5, -14.25)
  line L8 (42.5, -14.25) -> (42.5, -15.75)
  line L9 (42.5, -15.75) -> (44, -15.75)
  line L10 (44, -15.75) -> (44, -14.25)
  line L11 (44, -14.25) -> (42.5, -15.75) construction
  line L12 (42.5, -14.25) -> (44, -15.75) construction
  line L13 (44, -4.25) -> (42.5, -4.25)
  line L14 (42.5, -4.25) -> (42.5, -5.75)
  line L15 (42.5, -5.75) -> (44, -5.75)
  line L16 (44, -5.75) -> (44, -4.25)
  line L17 (44, -4.25) -> (42.5, -5.75) construction
  line L18 (42.5, -4.25) -> (44, -5.75) construction
  line L19 (43.25, -15.75) -> (43.25, -14.25)
  line L20 (43.25, -5.75) -> (43.25, -4.25)
  line L21 (44, -9.25) -> (42.5, -9.25)
  line L22 (42.5, -9.25) -> (42.5, -10.75)
  line L23 (42.5, -10.75) -> (44, -10.75)
  line L24 (44, -10.75) -> (44, -9.25)
  line L25 (44, -9.25) -> (42.5, -10.75) construction
  line L26 (42.5, -9.25) -> (44, -10.75) construction
  line L27 (0, -20) -> (1.515, -20)
  line L28 (21.4847, -20) -> (-7.7282, -20) projected
  line L29 (0, -10.75) -> (0, -9.25) projected
  line L30 (1.5075, -14.25) -> (0.0075, -14.25)
  line L31 (0.0075, -14.25) -> (0.0075, -15.75)
  line L32 (0.0075, -15.75) -> (1.5075, -15.75)
  line L33 (1.5075, -15.75) -> (1.5075, -14.25)
  line L34 (-7.7282, -15) -> (21.4847, -15) projected
  line L35 (1.5075, -14.25) -> (0.0075, -15.75) construction
  line L36 (0.0075, -14.25) -> (1.5075, -15.75) construction
  line L37 (1.5075, -9.25) -> (0.0075, -9.25)
  line L38 (0.0075, -9.25) -> (0.0075, -10.75)
  line L39 (0.0075, -10.75) -> (1.5075, -10.75)
  line L40 (1.5075, -10.75) -> (1.5075, -9.25)
  line L41 (1.5075, -9.25) -> (0.0075, -10.75) construction
  line L42 (0.0075, -9.25) -> (1.5075, -10.75) construction
  line L43 (0, -10.75) -> (2, -10.75) projected
  line L44 (1.5075, -4.25) -> (0.0075, -4.25)
  line L45 (0.0075, -4.25) -> (0.0075, -5.75)
  line L46 (0.0075, -5.75) -> (1.5075, -5.75)
  line L47 (1.5075, -5.75) -> (1.5075, -4.25)
  line L48 (1.5075, -4.25) -> (0.0075, -5.75) construction
  line L49 (0.0075, -4.25) -> (1.5075, -5.75) construction
  line L50 (43.25, -15) -> (43.25, -14.25)
  line L51 (0.7575, -15.75) -> (0.7575, -14.25)
  line L52 (0.7575, -10.75) -> (0.7575, -10)
  line L53 (0.7575, -5.75) -> (0.7575, -4.25)
  line L54 (43.25, -10.75) -> (43.25, -9.25)
  line L55 (43.25, -5.75) -> (43.25, -5)
  line L56 (0.7575, -4.25) -> (0.7575, -5.75)
  line L57 (0.7575, -9.25) -> (0.7575, -10)
  line L58 (0.7575, -15.75) -> (0.7575, -14.25)
  line L59 (0.7575, -10.75) -> (0.7575, -9.25)
  line L60 (0.7575, 0) -> (0.7575, -5.75)
  line L61 (0.7575, -9.25) -> (0.7575, -10)
  point P0 (-8, -20)
  point P1 (43.25, -10)
  point P2 (0.7575, -15)
  point P3 (0.7575, -5)
  dimension "d211" = 1.5
  dimension "d212" = 1.5
  dimension "d213" = 1.5
  dimension "d214" = 1.5
  dimension "d215" = 1.5
  dimension "d216" = 1.5
  dimension "d217" = 1.5
  dimension "d218" = 1.5
  constraints: 110 end point, 29 midpoint, 14 parallel, 10 vertical, 8 perpendicular, 6 horizontal, 6 point on line, 1 collinear, 1 other
  measures "d211" distance of L8.end L7.end
  measures "d212" distance of L14.end L13.end
  measures "d213" distance of L23.end L22.end
  measures "d214" distance of L22.end L21.end
  measures "d215" distance of L32.end L31.end
  measures "d216" distance of L31.end L30.end
  measures "d217" distance of L39.end L38.end
  measures "d218" distance of L46.end L45.end
extrude "Extrusion53" cut sketch "Sketch48" against normal blind 8
sketch "Sketch49" plane through (0, 0, 20) normal (0, 0, 1) x (1, 0, 0)
  line L0 (8, -8) -> (-21.6494, -8)
  line L1 (-21.6494, -8) -> (-21.6494, 18.45)
  line L2 (-21.6494, 18.45) -> (71.4783, 18.45)
  line L3 (71.4783, 18.45) -> (71.4783, -8)
  line L4 (71.4783, -8) -> (-21.6494, -8)
  point P0 (0, 0)
  constraints: 10 end point, 4 perpendicular, 1 horizontal, 1 point on line
extrude "Extrusion54" cut sketch "Sketch49" against normal through all
sketch "Sketch50" plane through (0, 0, 0) normal (0, 0, -1) x (-1, 0, 0)
  line L0 (-9.5, -8) -> (-8.0075, -8) projected
  line L1 (-52, -8) -> (-52, -14) projected
  line L2 (-8.0075, -8) -> (-52, -8)
  line L3 (-52, -8) -> (-52, -9)
  line L4 (-52, -9) -> (-8.0075, -9)
  line L5 (-8.0075, -9) -> (-8.0075, -8)
  point P0 (0, 0)
  dimension "d223" = 1
  constraints: 8 end point, 2 parallel, 1 horizontal, 1 perpendicular, 1 point on line
  measures "d223" distance of L3.end L2.end
extrude "Extrusion55" cut sketch "Sketch50" against normal through all
sketch "Sketch51" plane through (8, -14, 20) normal (0, -1, 0) x (1, 0, 0)
  line L0 (1.5075, -5.75) -> (1.5075, -4.25) projected
  line L1 (0.0075, -4.25) -> (1.5075, -4.25) projected
  line L2 (1.5075, -5.75) -> (0.0075, -5.75)
  line L3 (0.0075, -5.75) -> (0.0075, -4.25)
  line L4 (0.0075, -4.25) -> (1.5075, -4.25)
  line L5 (1.5075, -4.25) -> (1.5075, -5.75)
  line L6 (1.5075, -10.75) -> (1.5075, -9.25) projected
  line L7 (0.0075, -9.25) -> (1.5075, -9.25) projected
  line L8 (1.5075, -10.75) -> (0.0075, -10.75)
  line L9 (0.0075, -10.75) -> (0.0075, -9.25)
  line L10 (0.0075, -9.25) -> (1.5075, -9.25)
  line L11 (1.5075, -9.25) -> (1.5075, -10.75)
  line L12 (1.5075, -15.75) -> (1.5075, -14.25) projected
  line L13 (1.5075, -14.25) -> (0.0075, -14.25)
  line L14 (0.0075, -14.25) -> (0.0075, -15.75)
  line L15 (0.0075, -15.75) -> (1.5075, -15.75)
  line L16 (1.5075, -15.75) -> (1.5075, -14.25)
  line L17 (42.5, 0) -> (42.5, -4.25) projected
  line L18 (44, -5.75) -> (42.5, -5.75) projected
  line L19 (42.5, -4.25) -> (44, -4.25)
  line L20 (44, -4.25) -> (44, -5.75)
  line L21 (44, -5.75) -> (42.5, -5.75)
  line L22 (42.5, -5.75) -> (42.5, -4.25)
  line L23 (42.5, -5.75) -> (42.5, -9.25) projected
  line L24 (44, -10.75) -> (42.5, -10.75) projected
  line L25 (42.5, -9.25) -> (44, -9.25)
  line L26 (44, -9.25) -> (44, -10.75)
  line L27 (44, -10.75) -> (42.5, -10.75)
  line L28 (42.5, -10.75) -> (42.5, -9.25)
  line L29 (42.5, -14.25) -> (44, -14.25) projected
  line L30 (44, -15.75) -> (42.5, -15.75) projected
  line L31 (42.5, -14.25) -> (44, -14.25)
  line L32 (44, -14.25) -> (44, -15.75)
  line L33 (44, -15.75) -> (42.5, -15.75)
  line L34 (42.5, -15.75) -> (42.5, -14.25)
  point P0 (-8, -20)
  constraints: 48 end point, 12 parallel, 6 horizontal, 6 perpendicular, 1 point on line
extrude "Extrusion56" add sketch "Sketch51" against normal blind 7
sketch "Sketch52" plane through (52, -14, 20) normal (1, 0, 0) x (0, 0, -1)
  line L0 (10.75, 6) -> (10.75, 5) projected
  line L1 (9.25, 6) -> (9.25, 7) projected
  line L2 (10.75, 5) -> (9.25, 5)
  line L3 (9.25, 5) -> (9.25, 7)
  line L4 (9.25, 7) -> (10.75, 7)
  line L5 (10.75, 7) -> (10.75, 5)
  point P0 (20, 14)
  constraints: 8 end point, 2 parallel, 1 horizontal, 1 perpendicular
extrude "Extrusion57" cut sketch "Sketch52" against normal through all
sketch "Sketch53" plane through (8.0075, -9, 20) normal (1, 0, 0) x (0, 0, -1)
  line L0 (0, 0) -> (0, -3.5) projected
  line L1 (0, 1) -> (9.25, 1) projected
  line L2 (0, 0) -> (4.2425, 0)
  line L3 (4.2425, 0) -> (4.2425, 1)
  line L4 (4.2425, 1) -> (0, 1)
  line L5 (0, 1) -> (0, 0)
  line L6 (14.25, 0) -> (5.75, 0) projected
  line L7 (5.75, 0) -> (9.2459, 0)
  line L8 (9.2459, 0) -> (9.2459, 1)
  line L9 (9.2459, 1) -> (5.75, 1)
  line L10 (5.75, 1) -> (5.75, 0)
  line L11 (10.75, 0) -> (9.25, 0) projected
  line L12 (10.75, 1) -> (14.25, 1) projected
  line L13 (10.75, 0) -> (14.25, 0)
  line L14 (14.25, 0) -> (14.25, 1)
  line L15 (14.25, 1) -> (10.75, 1)
  line L16 (10.75, 1) -> (10.75, 0)
  line L17 (20, -5) -> (20, 1) projected
  line L18 (20, 0) -> (15.75, 0) projected
  line L19 (20, 1) -> (15.75, 1)
  line L20 (15.75, 1) -> (15.75, 0)
  line L21 (15.75, 0) -> (20, 0)
  line L22 (20, 0) -> (20, 1)
  point P0 (20, 9)
  constraints: 32 end point, 8 parallel, 4 horizontal, 4 perpendicular, 2 point on line
extrude "Extrusion58" cut sketch "Sketch53" against normal blind 10
sketch "Sketch54" plane through (8, -14, 0) normal (-1, 0, 0) x (0, 0, 1)
  point P0 (0, 14)
sketch "Sketch55" plane through (8, -14, 0) normal (-1, 0, 0) x (0, 0, 1)
  line L0 (20, 1.5) -> (20, 5) projected
  line L1 (20, 5) -> (0, 5)
  line L2 (0, 5) -> (0, 7.2002)
  line L3 (0, 7.2002) -> (20, 7.2002)
  line L4 (20, 7.2002) -> (20, 5)
  point P0 (0, 14)
  constraints: 8 end point, 2 parallel, 1 horizontal, 1 perpendicular
extrude "Extrusion59" cut sketch "Sketch55" against normal through all
sketch "Sketch56" plane through (50.5, -9, 0) normal (0, 1, 0) x (1, 0, 0)
  line L0 (-42.5, -20) -> (1.5, -20) projected
  line L1 (1.5, -20) -> (0, -20)
  line L2 (-1, -20) -> (-1, 0) projected
  line L3 (0.75, -20) -> (0.75, 0)
  line L4 (1.5, -20) -> (1.5, 0) projected
  line L5 (0.75, -20) -> (0.75, -10)
  circle A0 centre (0.75, -15) radius 0.75
  line L6 (0, -20) -> (0, 0) projected
  line L7 (0.75, -10) -> (0.75, 0)
  line L8 (1.5, 0) -> (-42.5, 0) projected
  circle A1 centre (0.75, -5) radius 0.75
  line L9 (-41, -15.75) -> (-41, -20) projected
  line L10 (-42.5, -20) -> (-41, -20)
  line L11 (-41, -20) -> (-41.75, -20)
  line L12 (-41.75, -20) -> (-41.75, 0)
  line L13 (-41.75, -10) -> (-41.75, -20)
  line L14 (-41.75, -10) -> (-41.75, 0)
  circle A2 centre (-41.75, -15) radius 0.75
  circle A3 centre (-41.75, -5) radius 0.75
  point P0 (-50.5, 0)
  dimension "d234" = 1.5
  dimension "d235" = 1.5
  dimension "d236" = 1.5
  dimension "d237" = 1.5
  constraints: 18 end point, 8 midpoint, 4 centre point, 3 perpendicular, 2 collinear, 1 horizontal, 1 parallel, 1 point on line, 1 tangent
  measures "d234" distance of L0.end L1.end
  measures "d235" diameter of A1
  measures "d236" diameter of A2
  measures "d237" diameter of A3
extrude "Extrusion60" add sketch "Sketch56" along normal blind 1.8 contours A2 L12 | L12 A2 | A0 L3 | A3 L12 | L12 A3 | L3 A0 | A1 L3 | A1 L3
sketch "Sketch57" plane through (8, -14, 0) normal (-1, 0, 0) x (0, 0, 1)
  line L0 (20, 2) -> (0, 2) projected
  line L1 (9.25, 5) -> (10.75, 5) projected
  line L2 (10, 5) -> (10, 1.5075)
  line L3 (9.25, 1.5075) -> (10.75, 1.5075) projected
  circle A0 centre (10, 3.2537) radius 1.5
  point P0 (0, 14)
  dimension "d240" = 3
  constraints: 3 midpoint, 2 end point, 1 centre point
  measures "d240" diameter of A0
extrude "Extrusion61" cut sketch "Sketch57" against normal blind 1.8
fillet "Fillet8" radius 1 1 edges at (50.5, -12.5, 10)
sketch "Sketch58" plane through (0, 0, 20) normal (0, 0, 1) x (1, 0, 0)
  line L0 (17.5, -12.5) -> (17, -12) projected
  line L1 (17.5, -12.5) -> (9.5, -12.5)
  line L2 (9.5, -12.5) -> (9.5, -12)
  line L3 (9.5, -12) -> (17.5, -12)
  line L4 (17.5, -12) -> (17.5, -12.5)
  line L5 (18.5, -9) -> (18.5, -12.5) projected
  line L6 (29.5, -12.5) -> (29, -12) projected
  line L7 (18.5, -12) -> (29.5, -12)
  line L8 (29.5, -12) -> (29.5, -12.5)
  line L9 (29.5, -12.5) -> (18.5, -12.5)
  line L10 (18.5, -12.5) -> (18.5, -12)
  line L11 (42.5, -9) -> (42.5, -12.5) projected
  line L12 (30.5, -12) -> (42.5, -12)
  line L13 (42.5, -12) -> (42.5, -12.5)
  line L14 (42.5, -12.5) -> (30.5, -12.5)
  line L15 (30.5, -12.5) -> (30.5, -12)
  line L16 (43.5, -9) -> (43.5, -12.5) projected
  arc A0 (49.5, -12.5) -> (50.5, -11.5) centre (49.5, -11.5) ccw projected
  line L17 (43.5, -12.5) -> (50.5, -12.5)
  line L18 (50.5, -12.5) -> (50.5, -11.5)
  line L19 (50.5, -11.5) -> (43.5, -11.5)
  line L20 (43.5, -11.5) -> (43.5, -12.5)
  point P0 (0, 0)
  constraints: 32 end point, 8 parallel, 4 horizontal, 4 perpendicular, 3 point on line
extrude "Extrusion62" cut sketch "Sketch58" against normal through all
sketch "Sketch59" plane through (9.5, -12.5, 20) normal (0, 1, 0) x (1, 0, 0)
  line L0 (42.5, 20) -> (-1.5, 20) projected
  line L1 (0.0241, 20) -> (4.0241, 20)
  line L2 (0, 9.25) -> (0, 5.75) projected
  line L3 (2.0241, 20) -> (2.0241, 0)
  line L4 (-1.5, 0) -> (42.5, 0) projected
  line L5 (2.0241, 20) -> (2.0241, 16)
  line L6 (2.0241, 20) -> (3.7562, 19)
  line L7 (3.7562, 19) -> (3.7562, 17)
  line L8 (3.7562, 17) -> (2.0241, 16)
  line L9 (2.0241, 16) -> (0.2921, 17)
  line L10 (0.2921, 17) -> (0.2921, 19)
  line L11 (0.2921, 19) -> (2.0241, 20)
  line L12 (3.2562, 18.7113) -> (2.0241, 19.4226)
  line L13 (2.0241, 19.4226) -> (0.7921, 18.7113)
  line L14 (0.7921, 18.7113) -> (0.7921, 17.2887)
  line L15 (0.7921, 17.2887) -> (2.0241, 16.5774)
  line L16 (2.0241, 16.5774) -> (3.2562, 17.2887)
  line L17 (3.2562, 17.2887) -> (3.2562, 18.7113)
  point P0 (-9.5, 20)
  point P1 (2.0241, 18)
  dimension "d246" = 4
  dimension "d247" = 4
  dimension "d248" = 0.5
  constraints: 30 end point, 4 point on line, 2 midpoint, 1 vertical, 18 other
  measures "d246" distance of L1.start L1.end
  measures "d247" distance of L3.start L5.end
  measures "d248" distance between parallel lines of L6 L12
extrude "Extrusion63" add sketch "Sketch59" along normal blind 0.5 contours L6 L7 L8 L3 L16 L17 L12 | L3 L13 L14 L15 L9 L10 L11
pattern_linear "Rectangular Pattern1" count 12 spacing 3.5 along (1, 0, 0) count 6 spacing 3.5 along (0, 0, 1) of "Extrusion63"
sketch "Sketch60" plane through (8, -14, 20) normal (0, -1, 0) x (1, 0, 0)
  line L0 (0, 0) -> (0, -20) projected
  line L1 (0, 0) -> (44.0811, 0)
  line L2 (44.0811, 0) -> (44.0811, 1.7426)
  line L3 (44.0811, 1.7426) -> (0, 1.7426)
  line L4 (0, 1.7426) -> (0, 0)
  point P0 (-8, -20)
  constraints: 8 end point, 2 parallel, 1 horizontal, 1 perpendicular
extrude "Extrusion64" cut sketch "Sketch60" against normal through all
body "Solid1"
